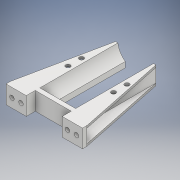
# Autodesk Inventor part: learnbotEncajeBateria
Saved by Autodesk Inventor 2017 (Build 210142000, 142)
## iProperties
Part Number: learnbotEncajeBateria
Material: Genérico
Document SubType Name: Modeling
Designer: rober
Density: 1 g/cm^3
Appearance: Valor por defecto
Author: rober
Autodesk Inventor part; units mm, degrees
ref_plane "YZ Plane" through (0, 0, 0) normal (1, 0, 0) x (0, 1, 0)
ref_plane "XZ Plane" through (0, 0, 0) normal (0, 1, 0) x (-1, 0, 0)
ref_plane "XY Plane" through (0, 0, 0) normal (0, 0, 1) x (1, 0, 0)
sketch "Boceto1" plane through (0, 0, 0) normal (0, 0, 1) x (1, 0, 0)
  line L0 (0, 0) -> (0, 0.3)
  line L1 (1.35, 0.9) -> (1.35, 11.3)
  line L2 (1.35, 11.3) -> (0, 0.3)
  line L3 (3.75, 0.9) -> (3.75, 11.3)
  line L4 (3.75, 11.3) -> (5.1, 0.3)
  line L5 (5.1, 0) -> (5.1, 0.3)
  line L6 (1.35, 0.9) -> (3.75, 0.9)
  line L7 (3.75, 0.6) -> (1.35, 0.6)
  line L8 (3.75, 0.6) -> (3.75, 0)
  line L9 (1.35, 0.6) -> (1.35, 0)
  line L10 (0, 0) -> (1.35, 0)
  line L11 (3.75, 0) -> (5.1, 0)
  line L12 (1.35, 11.3) -> (1.85, 11.3)
  line L13 (1.85, 11.3) -> (1.85, 0.9)
  line L14 (3.75, 11.3) -> (3.25, 11.3)
  line L15 (3.25, 11.3) -> (3.25, 0.9)
  constraints: 32 end point, 2 point on line
extrude "Extrusión1" add sketch "Boceto1" along normal blind 1.2 contours L0 L2 L1 L6 L3 L4 L5 L11 L8 L7 L9 L10
sketch "Boceto2" plane through (1.35, 0.9, 0) normal (0, 1, 0) x (1, 0, 0)
  line L0 (2.55, 0) -> (-0.15, 0)
  line L1 (-0.15, 0) -> (-0.15, -1.2)
  line L2 (-0.15, -1.2) -> (2.55, -1.2)
  line L3 (2.55, -1.2) -> (2.55, 0)
  line L4 (0, 0) -> (0, -1.2)
  line L5 (2.4, 0) -> (2.4, -1.2)
  line L6 (-0.15, -1.2) -> (-1.35, -1.2)
  line L7 (-1.35, -1.2) -> (-1.35, 0)
  line L8 (-1.35, 0) -> (-0.15, 0)
  line L9 (-0.15, 0) -> (-0.15, -0.15)
  line L10 (-0.15, -0.15) -> (-1.35, -0.15)
  line L11 (-1.35, -1.05) -> (-0.15, -1.05)
  line L12 (2.55, -1.2) -> (3.75, -1.2)
  line L13 (3.75, -1.2) -> (3.75, 0)
  line L14 (3.75, 0) -> (2.55, 0)
  line L15 (2.55, -0.15) -> (3.75, -0.15)
  line L16 (3.75, -1.05) -> (2.55, -1.05)
  line L17 (2.4, 0) -> (1.9, 0)
  line L18 (1.9, 0) -> (1.9, -0.15)
  line L19 (0, 0) -> (0.5, 0)
  line L20 (0.5, 0) -> (0.5, -0.15)
  arc A0 (2.3906, -1.2) -> (1.9, -0.3753) centre (1.2, -1.35) ccw
  line L21 (0, -1.2) -> (0.0094, -1.2)
  line L22 (0.5, -0.15) -> (0.5, -0.3753)
  line L23 (1.9, -0.15) -> (1.9, -0.3753)
  line L24 (2.4, -1.2) -> (2.3906, -1.2)
  arc A1 (0.5, -0.3753) -> (0.0094, -1.2) centre (1.2, -1.35) ccw
  line L25 (0, 0) -> (-1.35, 0) projected
  line L26 (-1.35, 0) -> (-1.35, -1.2) projected
  line L27 (0, -1.2) -> (-1.35, -1.2) projected
  line L28 (0, 0) -> (0, -1.2) projected
  line L29 (3.75, 0) -> (2.4, 0) projected
  line L30 (2.4, 0) -> (2.4, -1.2) projected
  line L31 (3.75, -1.2) -> (2.4, -1.2) projected
  line L32 (3.75, 0) -> (3.75, -1.2) projected
  line L33 (2.4, 0) -> (0, 0) projected
  line L34 (0, 0) -> (0, -1.2) projected
  line L35 (2.4, -1.2) -> (0, -1.2) projected
  line L36 (2.4, 0) -> (2.4, -1.2) projected
  constraints: 50 end point, 16 point on line, 4 point on circle, 2 centre point
extrude "Extrusión2" cut sketch "Boceto2" along normal blind 12 contours L15 L13 L16 L3 | L1 L11 L7 L10
sketch "Boceto3" plane through (1.35, 0.9, 0) normal (0, 1, 0) x (1, 0, 0)
  line L0 (2.55, 0) -> (-0.15, 0)
  line L1 (-0.15, 0) -> (-0.15, -1.2)
  line L2 (-0.15, -1.2) -> (2.55, -1.2)
  line L3 (2.55, -1.2) -> (2.55, 0)
  line L4 (0, 0) -> (0, -1.2)
  line L5 (2.4, 0) -> (2.4, -1.2)
  line L6 (-0.15, -1.2) -> (-1.35, -1.2)
  line L7 (-1.35, -1.2) -> (-1.35, 0)
  line L8 (-1.35, 0) -> (-0.15, 0)
  line L9 (-0.15, 0) -> (-0.15, -0.15)
  line L10 (-0.15, -0.15) -> (-1.35, -0.15)
  line L11 (-1.35, -1.05) -> (-0.15, -1.05)
  line L12 (2.55, -1.2) -> (3.75, -1.2)
  line L13 (3.75, -1.2) -> (3.75, 0)
  line L14 (3.75, 0) -> (2.55, 0)
  line L15 (2.55, -0.15) -> (3.75, -0.15)
  line L16 (3.75, -1.05) -> (2.55, -1.05)
  line L17 (2.4, 0) -> (1.9, 0)
  line L18 (1.9, 0) -> (1.9, -0.15)
  line L19 (0, 0) -> (0.5, 0)
  line L20 (0.5, 0) -> (0.5, -0.15)
  arc A0 (2.3906, -1.2) -> (1.9, -0.3753) centre (1.2, -1.35) ccw
  line L21 (0, -1.2) -> (0.0094, -1.2)
  line L22 (0.5, -0.15) -> (0.5, -0.3753)
  line L23 (1.9, -0.15) -> (1.9, -0.3753)
  line L24 (2.4, -1.2) -> (2.3906, -1.2)
  arc A1 (0.5, -0.3753) -> (0.0094, -1.2) centre (1.2, -1.35) ccw
  line L25 (0, 0) -> (-1.35, 0)
  line L26 (-1.35, 0) -> (-1.35, -1.2)
  line L27 (0, -1.2) -> (-1.35, -1.2)
  line L28 (0, 0) -> (0, -1.2)
  line L29 (3.75, 0) -> (2.4, 0)
  line L30 (2.4, 0) -> (2.4, -1.2)
  line L31 (3.75, -1.2) -> (2.4, -1.2)
  line L32 (3.75, 0) -> (3.75, -1.2)
  line L33 (2.4, 0) -> (0, 0)
  line L34 (0, 0) -> (0, -1.2)
  line L35 (2.4, -1.2) -> (0, -1.2)
  line L36 (2.4, 0) -> (2.4, -1.2)
  constraints: 74 end point, 16 point on line, 4 point on circle, 2 centre point
extrude "Extrusión3" add sketch "Boceto3" along normal blind 10.4 contours L5 L2 A0 L23 L18 L0 | L20 L22 A1 L2 L4 L0
sketch "Boceto4" plane through (1.35, 11.3, 0) normal (0, 1, 0) x (1, 0, 0)
  line L0 (0, 0) -> (0, -1.2) projected
  line L1 (0, -1.2) -> (0.0094, -1.2) projected
  arc A0 (0.5, -0.3753) -> (0.0094, -1.2) centre (1.2, -1.35) ccw projected
  line L2 (0.5, -0.3753) -> (0.5, 0) projected
  line L3 (0.5, 0) -> (0, 0) projected
  line L4 (2.4, 0) -> (1.9, 0) projected
  line L5 (1.9, 0) -> (1.9, -0.3753) projected
  arc A1 (2.3906, -1.2) -> (1.9, -0.3753) centre (1.2, -1.35) ccw projected
  line L6 (2.3906, -1.2) -> (2.4, -1.2) projected
  line L7 (2.4, 0) -> (2.4, -1.2) projected
  line L8 (2.55, 0) -> (-0.15, 0)
  line L9 (-0.15, 0) -> (-0.15, -1.2)
  line L10 (-0.15, -1.2) -> (2.55, -1.2)
  line L11 (2.55, -1.2) -> (2.55, 0)
  line L12 (0, 0) -> (0, -1.2)
  line L13 (2.4, 0) -> (2.4, -1.2)
  line L14 (-0.15, -1.2) -> (-1.35, -1.2)
  line L15 (-1.35, -1.2) -> (-1.35, 0)
  line L16 (-1.35, 0) -> (-0.15, 0)
  line L17 (-0.15, 0) -> (-0.15, -0.15)
  line L18 (-0.15, -0.15) -> (-1.35, -0.15)
  line L19 (-1.35, -1.05) -> (-0.15, -1.05)
  line L20 (2.55, -1.2) -> (3.75, -1.2)
  line L21 (3.75, -1.2) -> (3.75, 0)
  line L22 (3.75, 0) -> (2.55, 0)
  line L23 (2.55, -0.15) -> (3.75, -0.15)
  line L24 (3.75, -1.05) -> (2.55, -1.05)
  line L25 (2.4, 0) -> (1.9, 0)
  line L26 (1.9, 0) -> (1.9, -0.15)
  line L27 (0, 0) -> (0.5, 0)
  line L28 (0.5, 0) -> (0.5, -0.15)
  arc A2 (2.3906, -1.2) -> (1.9, -0.3753) centre (1.2, -1.35) ccw
  line L29 (0, -1.2) -> (0.0094, -1.2)
  line L30 (0.5, -0.15) -> (0.5, -0.3753)
  line L31 (1.9, -0.15) -> (1.9, -0.3753)
  line L32 (2.4, -1.2) -> (2.3906, -1.2)
  arc A3 (0.5, -0.3753) -> (0.0094, -1.2) centre (1.2, -1.35) ccw
  point P0 (-1.35, 0)
  constraints: 50 end point, 16 point on line, 4 point on circle, 2 centre point
extrude "Extrusión4" add sketch "Boceto4" against normal blind 10.4 contours L0 L10 L9 L8 | L8 L11 L10 L7
sketch "Boceto5" plane through (1.35, 11.3, 0) normal (0, 1, 0) x (1, 0, 0)
  line L0 (2.55, 0) -> (-0.15, 0)
  line L1 (-0.15, 0) -> (-0.15, -1.2)
  line L2 (-0.15, -1.2) -> (2.55, -1.2)
  line L3 (0, 0) -> (0, -1.2)
  line L4 (2.4, 0) -> (2.4, -1.2)
  line L5 (0, -1.2) -> (0.0094, -1.2)
  line L6 (0.5, -0.15) -> (0.5, -0.3753)
  line L7 (0, 0) -> (0.5, 0)
  line L8 (0.5, 0) -> (0.5, -0.15)
  arc A0 (0.5, -0.3753) -> (0.0094, -1.2) centre (1.2, -1.35) ccw
  line L9 (2.4, -1.2) -> (0, -1.2)
  line L10 (2.4, 0) -> (0, 0)
  line L11 (1.9, 0) -> (1.9, -0.15)
  line L12 (2.4, 0) -> (1.9, 0)
  line L13 (-0.15, -1.2) -> (-1.35, -1.2)
  line L14 (-1.35, -1.2) -> (-1.35, 0)
  line L15 (-1.35, 0) -> (-0.15, 0)
  line L16 (-0.15, 0) -> (-0.15, -0.15)
  line L17 (0, 0) -> (0, -1.2)
  line L18 (0, 0) -> (-1.35, 0)
  line L19 (-0.15, -0.15) -> (-1.35, -0.15)
  line L20 (-1.35, -1.05) -> (-0.15, -1.05)
  line L21 (-1.35, 0) -> (-1.35, -1.2)
  line L22 (0, -1.2) -> (-1.35, -1.2)
  line L23 (0, 0) -> (0, -1.2)
  line L24 (2.55, -1.2) -> (2.55, 0)
  line L25 (2.55, -1.2) -> (3.75, -1.2)
  line L26 (3.75, -1.2) -> (3.75, 0)
  line L27 (3.75, 0) -> (2.55, 0)
  line L28 (2.55, -0.15) -> (3.75, -0.15)
  line L29 (3.75, -1.05) -> (2.55, -1.05)
  line L30 (1.9, -0.15) -> (1.9, -0.3753)
  arc A1 (2.3906, -1.2) -> (1.9, -0.3753) centre (1.2, -1.35) ccw
  line L31 (2.4, -1.2) -> (2.3906, -1.2)
  line L32 (2.4, 0) -> (2.4, -1.2)
  line L33 (2.4, 0) -> (2.4, -1.2)
  line L34 (3.75, -1.2) -> (2.4, -1.2)
  line L35 (3.75, 0) -> (3.75, -1.2)
  line L36 (3.75, 0) -> (2.4, 0)
  constraints: 74 end point, 16 point on line, 4 point on circle, 2 centre point
extrude "Extrusión5" cut sketch "Boceto5" against normal blind 11 contours L28 L26 L29 L24 | L1 L20 L14 L19
sketch "Boceto6" plane through (1.35, 0.3, 0) normal (0, 1, 0) x (1, 0, 0)
  line L0 (2.55, 0) -> (-0.15, 0)
  line L1 (-0.15, 0) -> (-0.15, -1.2)
  line L2 (-0.15, -1.2) -> (2.55, -1.2)
  line L3 (2.55, -1.2) -> (2.55, 0)
  line L4 (0, 0) -> (0, -1.2)
  line L5 (2.4, 0) -> (2.4, -1.2)
  line L6 (-0.15, -1.2) -> (-1.35, -1.2)
  line L7 (-1.35, -1.2) -> (-1.35, 0)
  line L8 (-1.35, 0) -> (-0.15, 0)
  line L9 (-0.15, 0) -> (-0.15, -0.15)
  line L10 (-0.15, -0.15) -> (-1.35, -0.15)
  line L11 (-1.35, -1.05) -> (-0.15, -1.05)
  line L12 (2.55, -1.2) -> (3.75, -1.2)
  line L13 (3.75, -1.2) -> (3.75, 0)
  line L14 (3.75, 0) -> (2.55, 0)
  line L15 (2.55, -0.15) -> (3.75, -0.15)
  line L16 (3.75, -1.05) -> (2.55, -1.05)
  line L17 (2.4, 0) -> (1.9, 0)
  line L18 (1.9, 0) -> (1.9, -0.15)
  line L19 (0, 0) -> (0.5, 0)
  line L20 (0.5, 0) -> (0.5, -0.15)
  arc A0 (2.3906, -1.2) -> (1.9, -0.3753) centre (1.2, -1.35) ccw
  line L21 (0, -1.2) -> (0.0094, -1.2)
  line L22 (0.5, -0.15) -> (0.5, -0.3753)
  line L23 (1.9, -0.15) -> (1.9, -0.3753)
  line L24 (2.4, -1.2) -> (2.3906, -1.2)
  arc A1 (0.5, -0.3753) -> (0.0094, -1.2) centre (1.2, -1.35) ccw
  circle A2 centre (2.75, -0.6) radius 0.15
  circle A3 centre (3.35, -0.6) radius 0.15
  circle A4 centre (-0.35, -0.6) radius 0.15
  circle A5 centre (-0.95, -0.6) radius 0.15
  line L25 (-1.35, 0) -> (-1.35, -0.15) projected
  line L26 (-1.35, -0.15) -> (-1.35, -1.05) projected
  line L27 (-1.35, -1.05) -> (-1.35, -1.2) projected
  constraints: 50 end point, 16 point on line, 6 centre point, 4 point on circle
extrude "Extrusión6" cut sketch "Boceto6" against normal blind 10 contours A2 | A3 | A4 | A5
sketch "Boceto7" plane through (0, 0, 1.2) normal (0, 0, 1) x (1, 0, 0)
  line L0 (0, 0) -> (1.35, 0) projected
  line L1 (1.35, 0) -> (1.3594, 6.1)
  line L2 (1.3594, 0.9) -> (1.3594, 11.3) projected
  line L3 (1.3594, 6.1) -> (7.7947, 6.0901)
  line L4 (7.7947, 6.0901) -> (7.8047, 12.5901)
  line L5 (7.8047, 12.5901) -> (-2.1953, 12.6055)
  line L6 (-2.1953, 12.6055) -> (-2.2053, 6.1055)
  line L7 (-2.2053, 6.1055) -> (1.3594, 6.1)
  dimension "d12" = 6.1
  dimension "d13" = 6.5
  dimension "d14" = 10
  constraints: 12 end point, 5 perpendicular, 1 midpoint, 1 point on line
  measures "d12" distance of L0.end L1.end
  measures "d13" distance of L3.end L4.end
  measures "d14" distance of L4.end L5.end
extrude "Extrusión7" cut sketch "Boceto7" against normal blind 10
sketch "Boceto8" plane through (0, 0, 1.2) normal (0, 0, 1) x (1, 0, 0)
  line L0 (1.2, 6.1002) -> (1.2, 0.3) projected
  line L1 (3.9, 6.0961) -> (3.9, 0.3) projected
  line L2 (0, 0.3) -> (0, 0) projected
  line L3 (5.1, 0) -> (5.1, 0.3) projected
  line L4 (0, 0.3) -> (1.2, 6.1002)
  line L5 (1.2, 6.873) -> (1.2, 6.1002)
  line L6 (0, 0.3) -> (-0.3806, 0.3)
  line L7 (-0.3806, 0.3) -> (-0.3806, 6.873)
  line L8 (-0.3806, 6.873) -> (1.2, 6.873)
  line L9 (3.25, 0.9) -> (1.85, 0.9) projected
  line L10 (2.55, 0.9) -> (2.55, 4.8471)
  line L11 (3.9, 6.1002) -> (3.9, 0.3)
  line L12 (5.1, 0.3) -> (5.1, 0)
  line L13 (5.1, 0.3) -> (3.9, 6.1002)
  line L14 (3.9, 6.873) -> (3.9, 6.1002)
  line L15 (5.1, 0.3) -> (5.4806, 0.3)
  line L16 (5.4806, 0.3) -> (5.4806, 6.873)
  line L17 (5.4806, 6.873) -> (3.9, 6.873)
  constraints: 26 end point, 4 symmetric about line, 2 vertical, 1 horizontal, 1 midpoint, 1 parallel, 1 perpendicular
extrude "Extrusión8" cut sketch "Boceto8" against normal blind 10
sketch "Boceto9" plane through (0, 0, 1.2) normal (0, 0, 1) x (1, 0, 0)
  line L0 (0, 0) -> (0, 0.3)
  line L1 (1.35, 0.9) -> (1.35, 6.1)
  line L2 (1.2, 6.1) -> (0, 0.3)
  line L3 (3.75, 0.9) -> (3.75, 6.1)
  line L4 (3.9, 6.1) -> (5.1, 0.3)
  line L5 (5.1, 0) -> (5.1, 0.3)
  line L6 (1.35, 0.9) -> (3.75, 0.9)
  line L7 (3.75, 0.6) -> (1.35, 0.6)
  line L8 (3.75, 0.6) -> (3.75, 0)
  line L9 (1.35, 0.6) -> (1.35, 0)
  line L10 (0, 0) -> (1.35, 0)
  line L11 (3.75, 0) -> (5.1, 0)
  line L12 (1.85, 6.1) -> (1.85, 0.9)
  line L13 (3.25, 6.1) -> (3.25, 0.9)
  line L14 (1.2, 6.1) -> (1.85, 6.1)
  line L15 (3.25, 6.1) -> (3.75, 6.1)
  line L16 (1.35, 6.1) -> (1.2, 6.1)
  line L17 (3.75, 6.1) -> (3.9, 6.1)
  circle A0 centre (1.0336, 4) radius 0.15
  circle A1 centre (1.0336, 3.1) radius 0.15
  circle A2 centre (4.0664, 4) radius 0.15
  circle A3 centre (4.0664, 3.1) radius 0.15
  line L18 (1.35, 0.6) -> (3.75, 0.6) projected
  point P0 (0, 0)
  constraints: 36 end point, 4 centre point, 3 point on line
extrude "Extrusión9" cut sketch "Boceto9" against normal blind 0.5 contours A0 | A1 | A2 | A3
